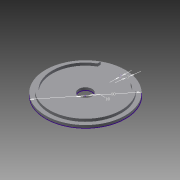
# Autodesk Inventor part: ServoHorn
Saved by Autodesk Inventor 2014 SP1 (Build 180222100, 222)
## iProperties
Created: 2015-03-17
Part Number: ServoHorn
Material: Generic
Document SubType Name: Modeling
Designer: Erin
Density: 1 g/cm^3
Appearance: Default
Author: Erin
Autodesk Inventor part; units mm, degrees
ref_plane "YZ Plane" through (0, 0, 0) normal (1, 0, 0) x (0, 1, 0)
ref_plane "XZ Plane" through (0, 0, 0) normal (0, 1, 0) x (-1, 0, 0)
sketch "Sketch1" plane through (0, 0, 0) normal (0, 0, 1) x (1, 0, 0)
  circle A0 centre (0, 0) radius 30
  circle A1 centre (0, 0) radius 27
  circle A2 centre (0, 0) radius 5
  circle A3 centre (0, 0) radius 25
  dimension "d0" = 60
  dimension "d1" = 3
  dimension "d2" = 10
  dimension "d3" = 2
  constraints: 4 centre point, 2 coincident
  measures "d0" diameter of A0
  measures "d1" radial gap between concentric circles of A1 A0
  measures "d2" diameter of A2
  measures "d3" radial gap between concentric circles of A3 A1
extrude "Extrusion1" add sketch "Sketch1" along normal blind 2 contours A0 | A1 | A3
extrude "Extrusion2" add sketch "Sketch1" along normal blind 4 contours A1
ref_plane "Work Plane1" through (0, 0, 2) normal (0, 0, 1) x (1, 0, 0)
sketch "Sketch2" plane through (0, 0, 2) normal (0, 0, 1) x (1, 0, 0)
  line L0 (-12.5, 32.3357) -> (12.5, 32.3357)
  line L1 (12.5, 32.3357) -> (12.5, 9.4484)
  line L2 (12.5, 9.4484) -> (-12.5, 9.4484)
  line L3 (-12.5, 9.4484) -> (-12.5, 32.3357)
  point P0 (0, 0)
  point P1 (0, 9.4484)
  dimension "d9" = 25
  constraints: 8 end point, 2 parallel, 1 horizontal, 1 midpoint, 1 perpendicular, 1 vertical alignment
  measures "d9" distance of L0.start L0.end
extrude "Extrusion3" cut sketch "Sketch2" along normal blind 4
body "Solid1"
